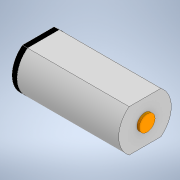
# Autodesk Inventor part: motor_051115
Saved by Autodesk Inventor 2021 (Build 250183000, 183)
## iProperties
Created: 2022-02-27
Part Number: motor_051115
Material: Generic
Document SubType Name: Modeling
Designer: ermoz
Density: 1 g/cm^3
Appearance: Default
Author: ermoz
Autodesk Inventor part; units mm, degrees
ref_plane "YZ Plane" through (0, 0, 0) normal (1, 0, 0) x (0, 1, 0)
ref_plane "XZ Plane" through (0, 0, 0) normal (0, 1, 0) x (-1, 0, 0)
ref_plane "XY Plane" through (0, 0, 0) normal (0, 0, 1) x (1, 0, 0)
sketch "Sketch1" plane through (0, 0, 0) normal (1, 0, 0) x (0, 1, 0)
  circle A0 centre (0, 0) radius 4.95
  line L0 (-3.95, -2.9833) -> (3.95, -2.9833)
  line L1 (3.95, -2.9833) -> (3.95, 2.9833)
  line L2 (3.95, 2.9833) -> (-3.95, 2.9833)
  line L3 (-3.95, 2.9833) -> (-3.95, -2.9833)
  line L4 (-3.95, -2.9833) -> (3.95, 2.9833) construction
  line L5 (3.95, -2.9833) -> (-3.95, 2.9833) construction
  dimension "d0" = 9.9
  dimension "d1" = 7.9
  constraints: 12 end point, 2 midpoint, 2 parallel, 1 coincident, 1 horizontal, 1 perpendicular, 3 other
  measures "d1" distance between parallel lines of L3 L1
extrude "Extrusion1" add sketch "Sketch1" along normal blind 19.1 contours L2 A0 | L1 L0 L3 L2 | A0 L0
sketch "Sketch2" plane through (19.1, 0, 0) normal (1, 0, 0) x (0, 0, -1)
  circle A0 centre (0, 0) radius 1.5
  dimension "d4" = 3
  constraints: 1 centre point, 1 coincident
  measures "d4" diameter of A0
extrude "Extrusion2" add sketch "Sketch2" along normal blind 0.4 separate body
sketch "Sketch3" plane through (0, 0, 0) normal (-1, 0, 0) x (0, 0, 1)
  line L0 (-2.9833, 3.95) -> (2.9833, 3.95) projected
  arc A0 (-2.9833, 3.95) -> (-2.9833, -3.95) centre (0, 0) ccw projected
  line L1 (2.9833, -3.95) -> (-2.9833, -3.95) projected
  arc A1 (2.9833, -3.95) -> (2.9833, 3.95) centre (0, 0) ccw projected
extrude "Extrusion3" add sketch "Sketch3" along normal blind 1 separate body
sketch "Sketch4" plane through (-1, 0, 0) normal (-1, 0, 0) x (0, 0, 1)
  circle A0 centre (0, 0) radius 1.5
  dimension "d9" = 3
  constraints: 1 centre point, 1 coincident
  measures "d9" diameter of A0
extrude "Extrusion4" add sketch "Sketch4" along normal blind 1 bodies 3
body "Solid1"
body "Solid2"
body "Solid3"
